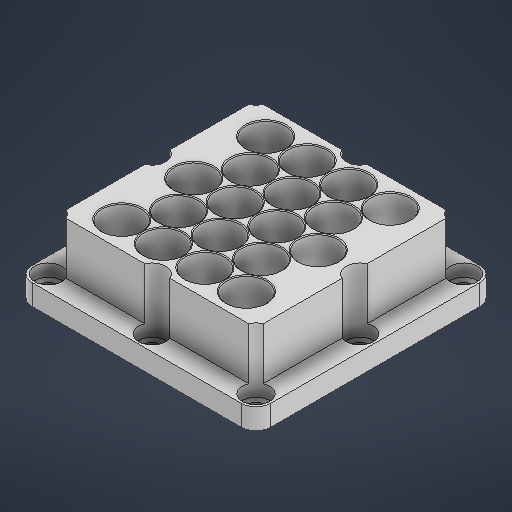
# Autodesk Inventor part: Battery Holder
Saved by Autodesk Inventor 2025 (Build 290162000, 162)
## iProperties
Created: 2025-08-08
Part Number: Battery Holder
Material: Generic
Document SubType Name: Modeling
Designer: mayhe
Density: 1 g/cm^3
Appearance: Default
Author: mayhe
Autodesk Inventor part; units mm, degrees
ref_plane "YZ Plane" through (0, 0, 0) normal (1, 0, 0) x (0, 1, 0)
ref_plane "XZ Plane" through (0, 0, 0) normal (0, 1, 0) x (-1, 0, 0)
ref_plane "XY Plane" through (0, 0, 0) normal (0, 0, 1) x (1, 0, 0)
sketch "Sketch1" plane through (0, 0, 0) normal (0, 1, 0) x (-1, 0, 0)
  line L0 (57.5, 57.5) -> (-57.5, 57.5)
  line L1 (-57.5, 57.5) -> (-57.5, -57.5)
  line L2 (-57.5, -57.5) -> (57.5, -57.5)
  line L3 (57.5, -57.5) -> (57.5, 57.5)
  line L4 (57.5, 57.5) -> (-57.5, -57.5) construction
  line L5 (-57.5, 57.5) -> (57.5, -57.5) construction
  point P0 (0, 0)
  dimension "d0" = 115
  dimension "d1" = 115
  constraints: 12 end point, 2 midpoint, 2 parallel, 1 horizontal, 1 perpendicular
  measures "d0" distance of L2.end L1.end
  measures "d1" distance of L1.end L0.end
extrude "Extrusion1" add sketch "Sketch1" along normal blind 10
sketch "Sketch4" plane through (0, 10, 0) normal (0, 1, 0) x (1, 0, 0)
  line L0 (-47.5, -47.5) -> (47.5, -47.5)
  line L1 (47.5, -47.5) -> (47.5, 47.5)
  line L2 (47.5, 47.5) -> (-47.5, 47.5)
  line L3 (-47.5, 47.5) -> (-47.5, -47.5)
  line L4 (-57.5, 57.5) -> (-57.5, -57.5) projected
  line L5 (-57.5, 0) -> (-47.5, 0)
  line L6 (-30, 34.641) -> (30, 34.641)
  line L7 (30, 34.641) -> (30, -34.641)
  line L8 (30, -34.641) -> (-30, -34.641)
  line L9 (-30, -34.641) -> (-30, 34.641)
  line L10 (-30, 34.641) -> (30, -34.641) construction
  line L11 (30, 34.641) -> (-30, -34.641) construction
  circle A0 centre (-30, 34.641) radius 9.5
  circle A1 centre (-10, 34.641) radius 9.5
  circle A2 centre (10, 34.641) radius 9.5
  circle A3 centre (30, 34.641) radius 9.5
  circle A4 centre (-30, 0) radius 9.5
  circle A5 centre (-10, 0) radius 9.5
  circle A6 centre (10, 0) radius 9.5
  circle A7 centre (30, 0) radius 9.5
  circle A8 centre (-30, -34.641) radius 9.5
  circle A9 centre (-10, -34.641) radius 9.5
  circle A10 centre (10, -34.641) radius 9.5
  circle A11 centre (30, -34.641) radius 9.5
  circle A12 centre (-20, 17.3205) radius 9.5
  circle A13 centre (0, 17.3205) radius 9.5
  circle A14 centre (20, 17.3205) radius 9.5
  circle A15 centre (-20, -17.3205) radius 9.5
  circle A16 centre (0, -17.3205) radius 9.5
  circle A17 centre (20, -17.3205) radius 9.5
  point P0 (47.3285, -94.6135)
  point P1 (-53.5957, 219.1108)
  point P2 (0, 0)
  dimension "d0" = 115
  dimension "d1" = 115
  dimension "d48" = 95
  dimension "d49" = 95
  dimension "d132" = 60
  dimension "d133" = 69.282
  dimension "d134" = 19
  dimension "d137" = 20
  dimension "d140" = 34.641
  dimension "d143" = 19
  dimension "d146" = 10
  dimension "d147" = 17.3205
  dimension "d150" = 20
  dimension "d153" = 34.641
  constraints: 22 end point, 18 centre point, 4 horizontal, 4 midpoint, 4 parallel, 2 perpendicular, 2 vertical, 1 coincident, 32 other
  measures "d48" distance of L2.end L1.end
  measures "d49" distance of L1.end L0.end
  measures "d132" distance of L7.end L8.end
  measures "d133" distance of L6.end L7.end
  measures "d134" diameter of A0
  measures "d137" distance of A0.centre A1.centre
  measures "d140" distance of A0.centre A4.centre
  measures "d143" diameter of A12
  measures "d146" horizontal distance of A1.centre A12.centre
  measures "d147" vertical distance of A12.centre A1.centre
  measures "d150" distance of A12.centre A13.centre
  measures "d153" distance of A12.centre A15.centre
extrude "Extrusion2" add sketch "Sketch4" along normal blind 25 contours L3 L2 L1 L0 | L6 A1 A2 A3 L7 A7 A11 L8 A10 A9 A8 L9 A4 A0
sketch "Sketch5" plane through (0, 35, 0) normal (0, 1, 0) x (1, 0, 0)
  line L0 (50, 50) -> (-50, 50)
  line L1 (-50, 50) -> (-50, -50)
  line L2 (-50, -50) -> (50, -50)
  line L3 (50, -50) -> (50, 50)
  line L4 (50, 50) -> (-50, -50) construction
  line L5 (-50, 50) -> (50, -50) construction
  circle A0 centre (-50, -50) radius 3.5
  circle A1 centre (0, -50) radius 3.5
  circle A2 centre (-50, 0) radius 3.5
  circle A3 centre (0, 0) radius 3.5
  circle A4 centre (50, -50) radius 3.5
  circle A5 centre (50, 0) radius 3.5
  circle A6 centre (-50, 50) radius 3.5
  circle A7 centre (0, 50) radius 3.5
  circle A8 centre (50, 50) radius 3.5
  point P0 (0, 0)
  dimension "d156" = 100
  dimension "d157" = 100
  dimension "d158" = 7
  dimension "d161" = 50
  dimension "d164" = 50
  constraints: 12 end point, 9 centre point, 2 horizontal, 2 midpoint, 2 parallel, 1 coincident, 1 perpendicular, 1 vertical, 16 other
  measures "d156" distance of L2.end L1.end
  measures "d157" distance of L1.end L0.end
  measures "d158" diameter of A0
  measures "d161" distance of A0.centre A1.centre
  measures "d164" distance of A0.centre A2.centre
hole "Hole3" at (-50, 35, 50) at (50, 35, 50) at (-50, 35, -50) at (50, 35, -50) at (-50, 35, 0) at (0, 35, 50) at (50, 35, 0) at (0, 35, -50) direction (0, -1, 0) diameter 7.125 end through all counterbore diameter 13 counterbore depth 31
fillet "Fillet1" radius 7.125 4 edges at (57.5, 5, 57.5) (57.5, 5, -57.5) (-57.5, 5, 57.5) (-57.5, 5, -57.5)
chamfer "Chamfer1" distance 0.4 angle 45 18 edges at (-39.5, 35, -34.641) (-19.5, 35, -34.641) (-29.5, 35, -17.3205) (0.5, 35, -34.641) (20.5, 35, -34.641) (10.5, 35, -17.3205) (-9.5, 35, -17.3205) (-39.5, 35, 0) (-19.5, 35, 0) (0.5, 35, 0) (20.5, 35, 0) (10.5, 35, 17.3205) (-9.5, 35, 17.3205) (-29.5, 35, 17.3205) (-39.5, 35, 34.641) (-19.5, 35, 34.641) (0.5, 35, 34.641) (20.5, 35, 34.641)
equation "\"d153\" = d124"
equation "\"d124\" = 34.641016"
body "Solid1"
